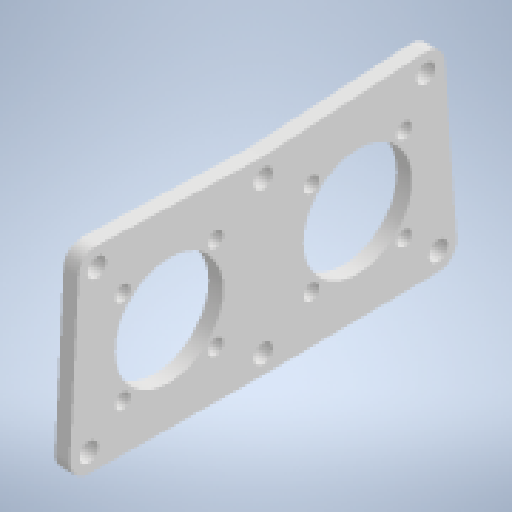
# Autodesk Inventor part: ChassiMotorMount3.0
Saved by Autodesk Inventor 2023 (Build 270158000, 158)
## iProperties
Created: 2022-09-16
Part Number: ChassiMotorMount3.0
Material: Generic
Document SubType Name: Modeling
Designer: deli
Density: 1 g/cm^3
Appearance: Default
Author: deli
Autodesk Inventor part; units mm, degrees
ref_plane "YZ Plane" through (0, 0, 0) normal (1, 0, 0) x (0, 1, 0)
ref_plane "XZ Plane" through (0, 0, 0) normal (0, 1, 0) x (-1, 0, 0)
ref_plane "XY Plane" through (0, 0, 0) normal (0, 0, 1) x (1, 0, 0)
sketch "Sketch1" plane through (0, 0, 0) normal (1, 0, 0) x (0, 1, 0)
  circle A0 centre (50.6472, 26.169) radius 2 projected
  circle A1 centre (17.4453, 27.9096) radius 2 projected
  circle A2 centre (33.1953, 10.8069) radius 7 construction
  circle A3 centre (49.3292, -9.2619) radius 2 projected
  circle A4 centre (17.0614, -9.2619) radius 2 projected
  circle A5 centre (17.4453, -46.4334) radius 2 projected
  circle A6 centre (51.3644, -43.8376) radius 2 projected
  circle A7 centre (33.1953, -29.3308) radius 7 construction
  arc A8 (54.6445, 26.0197) -> (50.8567, 30.1635) centre (50.6472, 26.169) ccw
  circle A9 centre (49.3292, -9.2619) radius 4 construction
  arc A10 (51.6696, -47.8259) -> (55.3574, -43.6009) centre (51.3644, -43.8376) ccw
  arc A11 (13.4455, -46.4747) -> (17.7505, -50.4217) centre (17.4453, -46.4334) ccw
  arc A12 (13.0633, -9.1382) -> (13.0616, -9.3032) centre (17.0614, -9.2619) ccw
  arc A13 (17.6547, 31.9041) -> (13.4455, 27.9508) centre (17.4453, 27.9096) ccw
  line L0 (13.4455, 27.9508) -> (13.0633, -9.1382)
  line L1 (13.0616, -9.3032) -> (13.4455, -46.4747)
  line L2 (50.8567, 30.1635) -> (17.6547, 31.9041)
  line L3 (51.6696, -47.8259) -> (17.7505, -50.4217)
  arc A14 (53.332, -9.1126) -> (53.3362, -9.4986) centre (57.3292, -9.2619) ccw
  line L4 (54.6445, 26.0197) -> (53.332, -9.1126)
  line L5 (55.3574, -43.6009) -> (53.3362, -9.4986)
  line L6 (17.0614, -9.2619) -> (57.3292, -9.2619) construction
  circle A15 centre (33.1953, 10.8069) radius 11.5
  circle A16 centre (33.1953, -29.3308) radius 11.5
  circle A17 centre (43.0948, 20.7064) radius 1.6
  circle A18 centre (43.0948, 0.9074) radius 1.6
  circle A19 centre (23.2958, 0.9074) radius 1.6
  circle A20 centre (23.2958, 20.7064) radius 1.6
  circle A21 centre (23.2958, -19.4313) radius 1.6
  circle A22 centre (43.0948, -19.4313) radius 1.6
  circle A23 centre (43.0948, -39.2303) radius 1.6
  circle A24 centre (23.2958, -39.2303) radius 1.6
  line L7 (43.0948, 20.7064) -> (43.0948, 0.9074) construction
  line L8 (43.0948, 0.9074) -> (23.2958, 0.9074) construction
  line L9 (23.2958, 0.9074) -> (23.2958, 20.7064) construction
  line L10 (23.2958, 20.7064) -> (43.0948, 20.7064) construction
  line L11 (43.0948, 20.7064) -> (23.2958, 0.9074) construction
  line L12 (23.2958, 20.7064) -> (43.0948, 0.9074) construction
  line L13 (43.0948, -19.4313) -> (43.0948, -39.2303) construction
  line L14 (43.0948, -39.2303) -> (23.2958, -39.2303) construction
  line L15 (23.2958, -39.2303) -> (23.2958, -19.4313) construction
  line L16 (23.2958, -19.4313) -> (43.0948, -19.4313) construction
  line L17 (23.2958, -39.2303) -> (43.0948, -19.4313) construction
  line L18 (23.2958, -19.4313) -> (43.0948, -39.2303) construction
  point P0 (0, 0)
  point P1 (53.5076, -16.7139)
  point P2 (49.3122, -19.5779)
  point P3 (21.0827, -58.3908)
  point P4 (33.1953, 10.8069)
  point P5 (33.1953, 10.8069)
  point P6 (33.1953, -29.3308)
  point P7 (19.3835, -56.016)
  point P8 (17.555, -42.4349)
  point P9 (17.3497, -15.1829)
  point P10 (53.615, -21.1734)
  point P11 (53.7299, -25.9433)
  point P12 (21.0179, -9.8497)
  point P13 (19.0255, -12.7465)
  dimension "d0" = 8
  dimension "d1" = 8
  dimension "d2" = 8
  dimension "d3" = 8
  dimension "d4" = 8
  dimension "d5" = 8
  dimension "d6" = 8
  dimension "d8" = 23
  dimension "d9" = 23
  dimension "d12" = 3.2
  dimension "d13" = 3.2
  dimension "d14" = 3.2
  dimension "d15" = 3.2
  dimension "d16" = 3.2
  dimension "d17" = 3.2
  dimension "d18" = 3.2
  dimension "d19" = 3.2
  dimension "d20" = 28
  dimension "d21" = 0
  dimension "d22" = 0
  dimension "d23" = 28
  constraints: 38 end point, 17 centre point, 12 point on circle, 12 tangent, 9 coincident, 6 perpendicular, 4 midpoint, 4 vertical, 1 horizontal, 1 point on line
  measures "d0" diameter of A8
  measures "d1" diameter of A13
  measures "d2" diameter of A12
  measures "d3" diameter of A9
  measures "d4" diameter of A10
  measures "d5" diameter of A11
  measures "d6" diameter of A14
  measures "d8" diameter of A15
  measures "d9" diameter of A16
  measures "d12" diameter of A17
  measures "d13" diameter of A18
  measures "d14" diameter of A19
  measures "d15" diameter of A20
  measures "d16" diameter of A21
  measures "d17" diameter of A22
  measures "d18" diameter of A23
  measures "d19" diameter of A24
  measures "d20" distance of L7.start L8.end
  measures "d21" distance of point (33.195, 10.807) A2.centre
  measures "d22" distance of A7.centre point (33.195, -29.331)
  measures "d23" distance of L14.end L13.start
extrude "Extrusion1" add sketch "Sketch1" along normal blind 3.175
equation "\"d1\" = d0"
equation "\"d2\" = d0"
equation "\"d3\" = d0"
equation "\"d4\" = d0"
equation "\"d5\" = d0"
equation "\"d6\" = d0"
equation "\"d9\" = d8"
equation "\"d13\" = d12"
equation "\"d14\" = d12"
equation "\"d15\" = d12"
equation "\"d16\" = d12"
equation "\"d17\" = d12"
equation "\"d18\" = d12"
equation "\"d19\" = d12"
equation "\"d23\" = d20"
body "Solid1"
